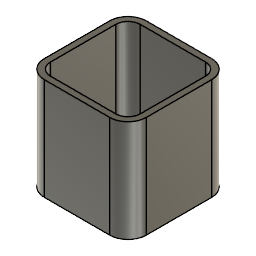
▢-100×100×6.0 (Autodesk Fusion 360 design; units mm, degrees)
Autodesk Fusion 360 part; units mm, degrees
sketch "スケッチ1" plane through (0, 0, 0) normal (0, 0, 1) x (1, 0, 0)
  line L0 (220.2952, 188.1753) -> (284.2952, 188.1753)
  line L1 (220.2952, 194.1753) -> (284.2952, 194.1753)
  line L2 (284.2952, 288.1753) -> (220.2952, 288.1753)
  line L3 (284.2952, 282.1753) -> (220.2952, 282.1753)
  arc A0 (220.2952, 288.1753) -> (202.2952, 270.1753) centre (220.2952, 270.1753) ccw
  arc A1 (220.2952, 282.1753) -> (208.2952, 270.1753) centre (220.2952, 270.1753) ccw
  line L4 (202.2952, 270.1753) -> (202.2952, 206.1753)
  line L5 (208.2952, 270.1753) -> (208.2952, 206.1753)
  arc A2 (202.2952, 206.1753) -> (220.2952, 188.1753) centre (220.2952, 206.1753) ccw
  arc A3 (208.2952, 206.1753) -> (220.2952, 194.1753) centre (220.2952, 206.1753) ccw
  arc A4 (302.2952, 270.1753) -> (284.2952, 288.1753) centre (284.2952, 270.1753) ccw
  arc A5 (296.2952, 270.1753) -> (284.2952, 282.1753) centre (284.2952, 270.1753) ccw
  line L6 (302.2952, 206.1753) -> (302.2952, 270.1753)
  line L7 (296.2952, 206.1753) -> (296.2952, 270.1753)
  arc A6 (284.2952, 188.1753) -> (302.2952, 206.1753) centre (284.2952, 206.1753) ccw
  arc A7 (284.2952, 194.1753) -> (296.2952, 206.1753) centre (284.2952, 206.1753) ccw
  point P0 (252.2952, 238.1753)
extrude "押し出し1" add sketch "スケッチ1" along normal blind 100
